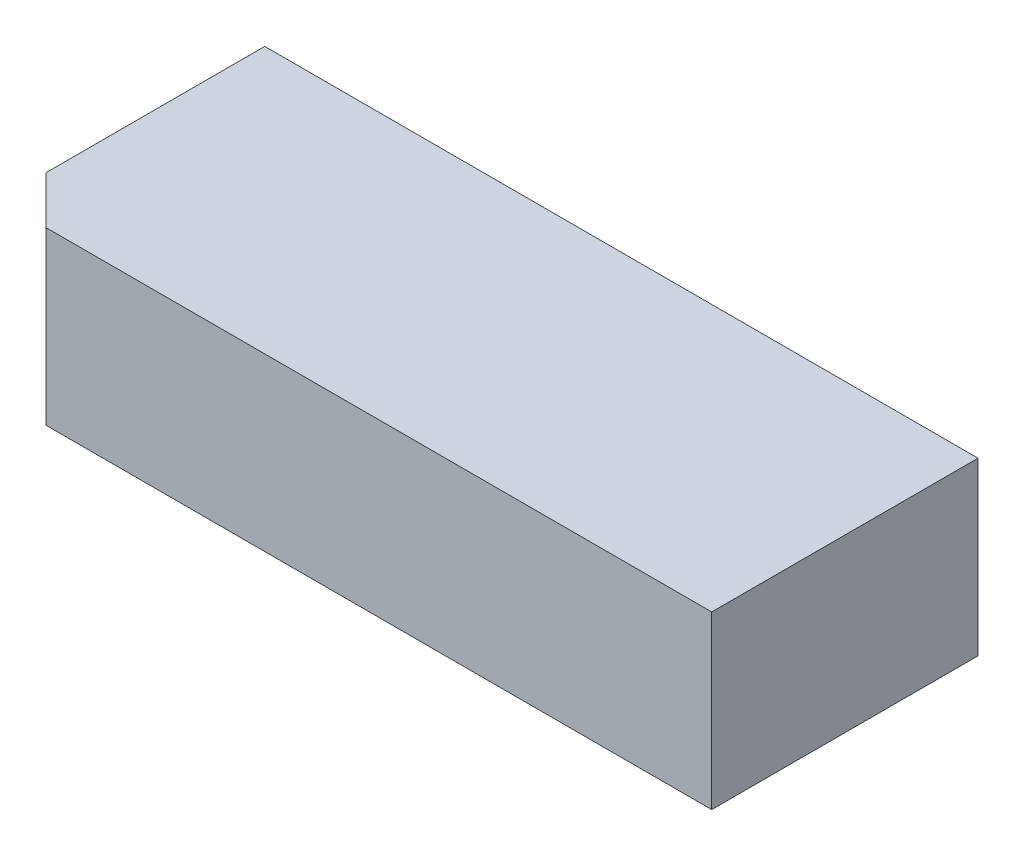
# Autodesk Inventor part: microswitch_cap
Saved by Autodesk Inventor 2025 (Build 290162000, 162)
## iProperties
Created: 2026-08-07
Part Number: microswitch_cap
Material: Типовые
Document SubType Name: Modeling
Designer: garin
Density: 1 g/cm^3
Appearance: По умолчанию
Author: garin
Autodesk Inventor part; units mm, degrees
ref_plane "YZ Plane" through (0, 0, 0) normal (1, 0, 0) x (0, 1, 0)
ref_plane "XZ Plane" through (0, 0, 0) normal (0, 1, 0) x (-1, 0, 0)
ref_plane "XY Plane" through (0, 0, 0) normal (0, 0, 1) x (1, 0, 0)
sketch "Эскиз1" plane through (0, 0, 0) normal (0, 1, 0) x (-1, 0, 0)
  line L0 (-7.5, 2.8) -> (7.5, 2.8)
  line L1 (7.5, 2.8) -> (7.5, -2.8)
  line L2 (7.5, -2.8) -> (-7.5, -2.8)
  line L3 (-7.5, -2.8) -> (-7.5, 2.8)
  line L4 (-7.5, 2.8) -> (7.5, -2.8) construction
  line L5 (7.5, 2.8) -> (-7.5, -2.8) construction
  point P0 (0, 0)
  dimension "d0" = 15
  dimension "d1" = 5.6
  constraints: 12 end point, 2 midpoint, 2 parallel, 1 horizontal, 1 perpendicular
  measures "d0" distance of L1.end L2.end
  measures "d1" distance of L0.end L1.end
extrude "Выдавливание1" add sketch "Эскиз1" along normal blind 3.6
chamfer "Фаска1" distance 1 angle 45 1 edges at (-7.5, 1.8, 2.8)
